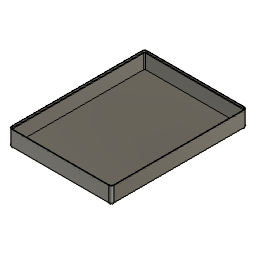
CDJ-Bottom-Tray (Autodesk Fusion 360 design; units mm, degrees)
Autodesk Fusion 360 part; units mm, degrees
sketch "Sketch1" plane through (0, 0, 0) normal (0, 0, 1) x (1, 0, 0)
  line L0 (0, 0) -> (324.3, 0)
  line L1 (324.3, 0) -> (324.3, 429.3)
  line L2 (324.3, 429.3) -> (0, 429.3)
  line L3 (0, 429.3) -> (0, 0)
  dimension "d7" = 324.3
  dimension "d8" = 429.3
  constraint horizontal L0
  constraint vertical L1
  constraint horizontal L2
  constraint vertical L3
  constraint coincident L0.start L3.end
  measures "d7" distance of L0.start L0.end
  measures "d8" distance of L0.start L2.end
extrude "Extrude1" add sketch "Sketch1" along normal blind 55
fillet "Fillet1" radius 8 4 edges at (324.3, 0, 27.5) (324.3, 429.3, 27.5) (0, 429.3, 27.5) (0, 0, 27.5)
shell "Shell1" thickness 5 removed faces 1 at (216.2, 283.5333, 55)
ref_plane "WorkPlane1" through (162.15, 214.65, 50) normal (0, 0, 1) x (1, 0, 0)
sketch "Sketch2" plane through (0, 0, 50) normal (0, 0, 1) x (1, 0, 0)
  line L0 (10, 427.3) -> (314.3, 427.3)
  line L1 (322.3, 419.3) -> (322.3, 10)
  line L2 (314.3, 2) -> (10, 2)
  line L3 (2, 10) -> (2, 419.3)
  arc A0 (8, 424.3) -> (5, 421.3) centre (8, 421.3) ccw
  line L4 (8, 424.3) -> (316.3, 424.3)
  arc A1 (319.3, 421.3) -> (316.3, 424.3) centre (316.3, 421.3) ccw
  line L5 (319.3, 421.3) -> (319.3, 8)
  arc A2 (316.3, 5) -> (319.3, 8) centre (316.3, 8) ccw
  line L6 (316.3, 5) -> (8, 5)
  arc A3 (5, 8) -> (8, 5) centre (8, 8) ccw
  line L7 (5, 8) -> (5, 421.3)
  arc A4 (0, 8) -> (8, 0) centre (8, 8) ccw
  line L8 (8, 0) -> (316.3, 0)
  arc A5 (316.3, 0) -> (324.3, 8) centre (316.3, 8) ccw
  line L9 (324.3, 8) -> (324.3, 421.3)
  arc A6 (324.3, 421.3) -> (316.3, 429.3) centre (316.3, 421.3) ccw
  line L10 (316.3, 429.3) -> (8, 429.3)
  arc A7 (8, 429.3) -> (0, 421.3) centre (8, 421.3) ccw
  line L11 (0, 421.3) -> (0, 8)
  arc A8 (2, 10) -> (10, 2) centre (10, 10) ccw
  arc A9 (10, 427.3) -> (2, 419.3) centre (10, 419.3) ccw
  arc A10 (322.3, 419.3) -> (314.3, 427.3) centre (314.3, 419.3) ccw
  arc A11 (314.3, 2) -> (322.3, 10) centre (314.3, 10) ccw
  dimension "d19" = 2
  dimension "d20" = 2
  dimension "d21" = 2
  dimension "d22" = 2
  dimension "d23" = 8
  constraint horizontal L0
  constraint vertical L1
  constraint horizontal L2
  constraint vertical L3
  constraint tangent L2 A8
  constraint tangent L3 A8
  constraint tangent L0 A9
  constraint tangent L3 A9
  constraint equal A8 A9
  constraint tangent L0 A10
  constraint tangent L1 A10
  constraint equal A8 A10
  constraint tangent L1 A11
  constraint tangent L2 A11
  constraint equal A8 A11
  measures "d19" distance of L1 L9
  measures "d20" distance of L0 L10
  measures "d21" distance of L3 L11
  measures "d22" distance of L2 L8
  measures "d23" radius of A8
extrude "Extrude2" cut sketch "Sketch2" along normal through all contours L0 L1 L2 L3 A8 A9 A10 A11
fillet "Fillet2" radius 8 1 faces at (216.2, 283.5333, 0)
equation "tray_depth = panel_depth + 2 * ( wall_thickness - lip_thickness ) + printer_tolerance"
equation "tray_width = panel_width + 2 * ( wall_thickness - lip_thickness ) + printer_tolerance"
equation "wall_height = 55 mm"
equation "wall_thickness = 2 mm + lip_thickness"
equation "corner_radius = 8 mm"
equation "lip_depth = 5 mm"
equation "d7 = tray_width"
equation "d8 = tray_depth"
equation "d9 = wall_height"
equation "d12 = corner_radius"
equation "d13 = wall_thickness"
equation "panel_width = 320 mm"
equation "panel_depth = 425 mm"
equation "lip_thickness = 3 mm"
equation "printer_tolerance = 0.3 mm"
equation "d18 = -lip_depth"
equation "d19 = wall_thickness - lip_thickness"
equation "d20 = wall_thickness - lip_thickness"
equation "d21 = wall_thickness - lip_thickness"
equation "d22 = wall_thickness - lip_thickness"
equation "d23 = corner_radius"
equation "d26 = corner_radius"
